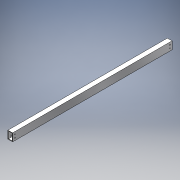
# Autodesk Inventor part: 前後機構_角柱1
Saved by Autodesk Inventor 2019.4 (Build 234330000, 330)
## iProperties
Created: 2021-12-05
Part Number: 前後機構_角柱1
Material: アルミニウム 6061
Document SubType Name: Modeling
Designer: 堀川皓史
Density: 2.7 g/cm^3
Appearance: アルミニウム - フラット
Author: 堀川皓史
Autodesk Inventor part; units mm, degrees
ref_plane "YZ Plane" through (0, 0, 0) normal (1, 0, 0) x (0, 1, 0)
ref_plane "XZ Plane" through (0, 0, 0) normal (0, 1, 0) x (-1, 0, 0)
ref_plane "XY Plane" through (0, 0, 0) normal (0, 0, 1) x (1, 0, 0)
sketch "スケッチ1" plane through (0, 0, 0) normal (0, 0, 1) x (1, 0, 0)
  line L0 (7.5, 12.5) -> (-7.5, 12.5)
  line L1 (-7.5, 12.5) -> (-7.5, -12.5)
  line L2 (-7.5, -12.5) -> (7.5, -12.5)
  line L3 (7.5, -12.5) -> (7.5, 12.5)
  line L4 (7.5, 12.5) -> (-7.5, -12.5) construction
  line L5 (-7.5, 12.5) -> (7.5, -12.5) construction
  line L6 (-5.5, 10.5) -> (5.5, 10.5)
  line L7 (5.5, 10.5) -> (5.5, -10.5)
  line L8 (5.5, -10.5) -> (-5.5, -10.5)
  line L9 (-5.5, -10.5) -> (-5.5, 10.5)
  point P0 (0, 0)
  dimension "d0" = 15
  dimension "d1" = 25
  dimension "d2" = 2
  constraints: 20 end point, 4 parallel, 2 midpoint, 2 perpendicular, 1 horizontal, 3 other
  measures "d0" distance of L2.end L1.end
  measures "d1" distance of L1.end L0.end
  measures "d2" distance between parallel lines of L0 L6
extrude "押し出し1" add sketch "スケッチ1" along normal blind 512
sketch "スケッチ2" plane through (7.5, -12.5, 0) normal (1, 0, 0) x (0, 0, -1)
  circle A0 centre (-7, 17.5) radius 1.6
  circle A1 centre (-7, 7.5) radius 1.6
  circle A2 centre (-505, 17.5) radius 1.6
  circle A3 centre (-505, 7.5) radius 1.6
  line L0 (-512, 0) -> (-512, 25) projected
  line L1 (0, 25) -> (-512, 25) projected
  line L2 (0, 0) -> (-512, 0) projected
  line L3 (0, 0) -> (0, 25) projected
  dimension "d7" = 3.2
  dimension "d8" = 3.2
  dimension "d13" = 3.2
  dimension "d14" = 3.2
  dimension "d17" = 10
  dimension "d23" = 7
  dimension "d24" = 7.5
  dimension "d25" = 10
  dimension "d26" = 7.5
  dimension "d27" = 7
  constraints: 4 centre point, 2 vertical alignment
  measures "d7" diameter of A0
  measures "d8" diameter of A1
  measures "d13" diameter of A2
  measures "d14" diameter of A3
  measures "d17" distance of A3.centre A2.centre
  measures "d23" distance from line of L0 A3.centre
  measures "d24" distance from line of L2 A3.centre
  measures "d25" distance of A1.centre A0.centre
  measures "d26" distance from line of L2 A1.centre
  measures "d27" distance from line of L3 A1.centre
extrude "押し出し2" cut sketch "スケッチ2" against normal through all contours A0 | A1 | A2 | A3
